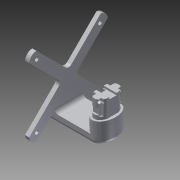
# Autodesk Inventor part: monitor-mount
Saved by Autodesk Inventor 2015 (Build 190159000, 159)
## iProperties
Created: 2015-03-06
Part Number: monitor-mount
Material: ABS Plastic
Document SubType Name: Modeling
Designer: Jody
Density: 1.06 g/cm^3
Appearance: Smooth - White
Mass: 59.874 g
Surface Area: 171.606 cm^2
Volume: 56.4849 cm^3
Author: Jody
Autodesk Inventor part; units mm, degrees
ref_plane "YZ Plane" through (0, 0, 0) normal (1, 0, 0) x (0, 1, 0)
ref_plane "XZ Plane" through (0, 0, 0) normal (0, 1, 0) x (-1, 0, 0)
ref_plane "XY Plane" through (0, 0, 0) normal (0, 0, 1) x (1, 0, 0)
sketch "Sketch1" plane through (0, 0, 0) normal (0, 1, 0) x (-1, 0, 0)
  ellipse E0 centre (0, 0) end of major axis (0, -16.9) minor radius 10.95
  dimension "d0" = 16.9
  dimension "d1" = 10.95
  constraints: 1 coincident, 2 other
extrude "Extrusion1" add sketch "Sketch1" along normal blind 25
sketch "Sketch2" plane through (0, 25, 0) normal (0, 1, 0) x (1, 0, 0)
  line L0 (7.6, 6.869) -> (7.6, -6.8693)
  line L1 (-7.6, -6.8693) -> (-7.6, 6.869)
  line L2 (1.547, -14.35) -> (-1.547, -14.35)
  line L3 (-1.547, 14.35) -> (1.547, 14.35)
  spline S0 degree 5 poles (7.6, 6.869) (7.3339, 7.69) (6.6747, 9.389) (5.6155, 11.3113) (4.2798, 12.863) (2.8086, 13.8602) (1.8557, 14.2496) (1.547, 14.35) knots 0 0 0 0 0 0 0.371815 0.797909 1 1 1 1 1 1
  line L4 (7.9552, 5.7734) -> (7.2448, 7.9647) construction
  arc A0 (7.863, 5.9868) -> (7.2954, 7.7378) centre (-10.8296, 0.8944) ccw construction
  spline S1 degree 5 poles (-1.547, 14.35) (-1.8557, 14.2496) (-2.8086, 13.8602) (-4.2798, 12.863) (-5.6155, 11.3113) (-6.6747, 9.389) (-7.3339, 7.69) (-7.6, 6.869) knots 0 0 0 0 0 0 0.202091 0.628185 1 1 1 1 1 1
  line L5 (-7.2448, 7.9647) -> (-7.9552, 5.7734) construction
  arc A1 (-7.2954, 7.7378) -> (-7.863, 5.9868) centre (10.8296, 0.8944) ccw construction
  spline S2 degree 5 poles (-7.6, -6.8693) (-7.3341, -7.6901) (-6.733, -9.2397) (-5.6943, -11.1801) (-4.3754, -12.7614) (-2.913, -13.7987) (-1.9626, -14.2149) (-1.547, -14.35) knots 0 0 0 0 0 0 0.37178 0.727887 1 1 1 1 1 1
  spline S3 degree 5 poles (1.547, -14.35) (1.9626, -14.2149) (2.913, -13.7987) (4.3754, -12.7614) (5.6943, -11.1801) (6.733, -9.2397) (7.3341, -7.6901) (7.6, -6.8693) knots 0 0 0 0 0 0 0.272113 0.62822 1 1 1 1 1 1
  line L6 (-2.5566, -14.0218) -> (-0.5374, -14.6782) construction
  arc A2 (-2.3246, -14.0283) -> (-0.7288, -14.5471) centre (0.1247, -9.2081) ccw construction
  line L7 (0.5374, -14.6782) -> (2.5566, -14.0218) construction
  arc A3 (0.7288, -14.5471) -> (2.3246, -14.0283) centre (-0.1247, -9.2081) ccw construction
  point P0 (5.4887, -11.1759)
  point P1 (2.672, 13.8453)
  point P2 (-5.4887, 11.1759)
  point P3 (-2.672, -13.8453)
  constraints: 24 end point, 8 midpoint, 4 centre point, 4 point on circle, 2 parallel, 1 horizontal, 1 perpendicular, 24 other
extrude "Extrusion3" add sketch "Sketch2" along normal blind 21
sketch "Sketch6" plane through (0, 46, 0) normal (0, 1, 0) x (1, 0, 0)
  line L0 (3.7, -9.8) -> (10.95, -9.8)
  line L1 (-10.95, -8.35) -> (-3.7, -8.35)
  line L2 (-3.7, -8.35) -> (-3.7, -16.9)
  line L3 (3.7, -9.8) -> (3.7, -16.9)
  line L4 (-3.7, -16.9) -> (-10.95, -8.35)
  line L5 (3.7, -16.9) -> (10.95, -9.8)
  line L6 (3.7, 9.8) -> (10.95, 9.8)
  line L7 (-10.95, 8.35) -> (-3.7, 8.35)
  line L8 (-3.7, 8.35) -> (-3.7, 16.9)
  line L9 (3.7, 9.8) -> (3.7, 16.9)
  line L10 (-3.7, 16.9) -> (-10.95, 8.35)
  line L11 (3.7, 16.9) -> (10.95, 9.8)
  point P0 (0, 0)
  constraints: 24 end point
extrude "Extrusion4" cut sketch "Sketch6" against normal blind 17.7
sketch "Sketch7" plane through (0, 46, 0) normal (0, 1, 0) x (1, 0, 0)
  ellipse E0 centre (0, 0) end of major axis (0, -16.9) minor radius 10.95 projected
  line L0 (10.581, -4.35) -> (-10.581, -4.35)
  line L1 (-10.581, -4.35) -> (-10.581, 4.35)
  line L2 (-10.581, 4.35) -> (10.581, 4.35)
  line L3 (10.581, 4.35) -> (10.581, -4.35)
  line L4 (10.581, -4.35) -> (-10.581, 4.35) construction
  line L5 (-10.581, -4.35) -> (10.581, 4.35) construction
  dimension "d23" = 8.7
  constraints: 12 end point, 2 midpoint, 2 parallel, 1 horizontal, 1 perpendicular, 2 other
  measures "d23" distance of L0.end L1.end
extrude "Extrusion5" cut sketch "Sketch7" against normal blind 2.4 contours L0 L1 L2 L3
sketch "Sketch8" plane through (7.6, 25, 6.8693) normal (1, 0, 0) x (0, 0, -1)
  line L0 (-7.4807, 4.8) -> (-7.4807, 12.1)
  line L1 (-5.4807, 4.8) -> (-5.4807, 12.1)
  line L2 (-7.4807, 4.8) -> (-5.4807, 4.8)
  line L3 (-5.4807, 12.1) -> (-7.4807, 12.1)
  line L4 (21.2193, 4.8) -> (21.2193, 12.1)
  line L5 (19.2193, 4.8) -> (19.2193, 12.1)
  line L6 (21.2193, 4.8) -> (19.2193, 4.8)
  line L7 (19.2193, 12.1) -> (21.2193, 12.1)
  point P0 (6.8693, -25)
  point P1 (0, 0)
  constraints: 16 end point, 2 horizontal
extrude "Extrusion6" cut sketch "Sketch8" against normal up to next
sketch "Sketch9" plane through (-7.6, 25, -6.869) normal (-1, 0, 0) x (0, 0, 1)
  line L0 (3.4692, 5) -> (10.2692, 5)
  line L1 (3.4692, 5) -> (3.4692, 18.6)
  line L2 (10.2692, 5) -> (10.2692, 18.6)
  line L3 (3.4692, 18.6) -> (10.2692, 18.6)
  point P0 (6.869, -25)
  constraints: 8 end point, 1 perpendicular
extrude "Extrusion7" cut sketch "Sketch9" against normal blind 3.5
sketch "Sketch10" plane through (-7.6, 30, -3.3999) normal (0, 0, 1) x (1, 0, 0)
  line L0 (0, 0) -> (3.5, 7.1937)
  line L1 (3.5, 0) -> (3.5, 13.6) projected
  line L2 (3.5, 7.1937) -> (3.5, 8.6937)
  line L3 (3.5, 8.6937) -> (0.864, 10.4946)
  line L4 (0, 0) -> (3.5, 0)
  line L5 (0, 0) -> (3.5, 0) projected
  line L6 (0.864, 10.4946) -> (3.5, 13.6)
  point P0 (7.6, -30)
  dimension "d36" = 8
  dimension "d37" = 1.5
  constraints: 10 end point, 2 point on line, 1 collinear
  measures "d36" distance of L0.start L0.end
  measures "d37" distance of L0.end L2.end
extrude "Extrusion8" add sketch "Sketch10" along normal up to next
fillet "Fillet1" radius 0.5 1 edges at (-6.736, 40.4946, 0.0001)
sketch "Sketch11" plane through (3.7, 46, 13.1272) normal (1, 0, 0) x (0, 0, -1)
  circle A0 centre (1.6989, -3.0978) radius 2.25
  line L0 (17.4772, -2.4) -> (8.7772, -2.4) projected
  line L1 (16.5271, -2.4) -> (9.7271, -2.4) projected
  circle A1 centre (24.5552, -3.0978) radius 2.25
  point P0 (13.1272, -46)
  dimension "d43" = 4.5
  constraints: 2 centre point
  measures "d43" diameter of A0
extrude "Extrusion9" cut sketch "Sketch11" along normal blind 10 and the other way blind 5
sketch "Sketch12" plane through (0, 0, 0) normal (0, -1, 0) x (1, 0, 0)
  ellipse E0 centre (0, 0) end of major axis (0, 16.9) minor radius 10.95 projected
  line L0 (0, 16.9) -> (0, -16.9)
  line L1 (0, -16.9) -> (-50, -16.9)
  line L2 (-50, -16.9) -> (-50, 16.9)
  line L3 (-50, 16.9) -> (0, 16.9)
  dimension "d50" = 50
  constraints: 8 end point, 2 parallel, 1 perpendicular, 1 vertical, 3 other
  measures "d50" distance of L0.end L1.end
extrude "Extrusion10" add sketch "Sketch12" against normal blind 10 contours E0 L1 L2 L3
sketch "Sketch13" plane through (-50, 0, -16.9) normal (-1, 0, 0) x (0, 0, 1)
  circle A0 centre (54.4, 75.1899) radius 2.25
  line L0 (25.3853, 37.6899) -> (63.569, 75.8737)
  line L1 (16.9, 46.1752) -> (55.0838, 84.359)
  arc A1 (63.569, 75.8737) -> (55.0838, 84.359) centre (54.4, 75.1899) ccw
  circle A2 centre (-20.6, 75.1899) radius 2.25
  line L2 (16.9, 46.1752) -> (-21.2838, 84.359)
  line L3 (8.4147, 37.6899) -> (-29.769, 75.8737)
  arc A3 (-21.2838, 84.359) -> (-29.769, 75.8737) centre (-20.6, 75.1899) ccw
  circle A4 centre (54.4, 75.1899) radius 2.25
  line L4 (8.4147, 37.6899) -> (-29.769, -0.4938)
  line L5 (16.9, 29.2046) -> (-21.2838, -8.9791)
  arc A5 (-29.769, -0.4938) -> (-21.2838, -8.9791) centre (-20.6, 0.1899) ccw
  circle A6 centre (54.4, 0.1899) radius 2.25
  line L6 (16.9, 29.2046) -> (55.0838, -8.9791)
  line L7 (25.3853, 37.6899) -> (63.569, -0.4938)
  arc A7 (55.0838, -8.9791) -> (63.569, -0.4938) centre (54.4, 0.1899) ccw
  circle A8 centre (-20.6, 0.1899) radius 2.25
  point P0 (16.9, 37.6899)
  point P1 (16.9, 37.6899)
  point P2 (16.9, 37.6899)
  point P3 (16.9, 37.6899)
  dimension "d58" = 4.5
  dimension "d63" = 4.5
  dimension "d64" = 4.5
  dimension "d65" = 4.5
  dimension "d66" = 4.5
  dimension "d67" = 75
  dimension "d68" = 75
  constraints: 16 end point, 9 centre point, 8 point on circle, 3 coincident
  measures "d58" diameter of A0
  measures "d63" diameter of A2
  measures "d64" diameter of A4
  measures "d65" diameter of A6
  measures "d66" diameter of A8
  measures "d67" distance of A0.centre A2.centre
  measures "d68" distance of A6.centre A1.centre
extrude "Extrusion11" add sketch "Sketch13" against normal blind 5
fillet "Fillet2" radius 5 4 edges at (-47.5, 46.1752, 0) (-47.5, 29.2046, 0) (-47.5, 37.6899, -8.4853) (-47.5, 37.6899, 8.4853)
sketch "Sketch14" plane through (0, 10, 0) normal (0, 1, 0) x (1, 0, 0)
  line L0 (-45, -16.9) -> (-50, -16.9)
  line L1 (-45, 16.9) -> (-45, -16.9)
  line L2 (-45, 16.9) -> (-50, 16.9)
  line L3 (-50, 16.9) -> (-50, -16.9)
  point P0 (0, 0)
  point P1 (-50, 14.2046)
  constraints: 8 end point, 2 horizontal, 2 point on line, 1 perpendicular
extrude "Extrusion12" add sketch "Sketch14" along normal up to next
fillet "Fillet4" radius 5 3 edges at (10.95, 0, 0) (-25, 0, 16.9) (-25, 0, -16.9)
fillet "Fillet5" radius 5 1 edges at (-45, 10, 0)
sketch "Sketch17" plane through (0, 0, 0) normal (0, -1, 0) x (1, 0, 0)
  line L0 (-44, 8.3852) -> (-4.0506, 8.3852) construction
  line L1 (-4.0506, 8.3852) -> (-4.0506, 4) construction
  line L2 (-4.0506, 4) -> (-44, 4) construction
  line L3 (-44, 4) -> (-44, 8.3852) construction
  line L4 (-44, -4.4007) -> (0.0705, -4.4007) construction
  line L5 (0.0705, -4.4007) -> (0.0705, -7.9) construction
  line L6 (0.0705, -7.9) -> (-44, -7.9) construction
  line L7 (-44, -7.9) -> (-44, -4.4007) construction
  line L8 (-50, 11.9) -> (-50, -11.9) projected
  line L9 (0, -11.9) -> (-50, -11.9) projected
  line L10 (-50, 3.5355) -> (-50, -3.5355) projected
  line L11 (-41.6175, 4.7292) -> (-42.06, 4.7292)
  line L12 (-42.06, 4.7292) -> (-42.06, 6.2268)
  spline S0 degree 2 poles (-42.06, 6.2268) (-42.06, 6.4083) (-42.094, 6.7203) (-42.1451, 6.8139) knots 0 0 0 1 2 2 2
  spline S1 degree 2 poles (-42.1451, 6.8139) (-42.1989, 6.9132) (-42.3918, 7.0096) (-42.5563, 7.0096) knots 0 0 0 1 2 2 2
  spline S2 degree 2 poles (-42.5563, 7.0096) (-42.7208, 7.0096) (-43.0697, 6.8338) (-43.237, 6.6919) knots 0 0 0 1 2 2 2
  line L13 (-43.237, 6.6919) -> (-43.237, 4.7292)
  line L14 (-43.237, 4.7292) -> (-43.6795, 4.7292)
  line L15 (-43.6795, 4.7292) -> (-43.6795, 8.3852)
  line L16 (-43.6795, 8.3852) -> (-43.237, 8.3852)
  line L17 (-43.237, 8.3852) -> (-43.237, 7.0635)
  spline S3 degree 2 poles (-43.237, 7.0635) (-43.0385, 7.2422) (-42.6556, 7.4294) (-42.44, 7.4294) knots 0 0 0 1 2 2 2
  spline S4 degree 2 poles (-42.44, 7.4294) (-42.0543, 7.4294) (-41.6175, 6.9188) (-41.6175, 6.4338) knots 0 0 0 1 2 2 2
  line L18 (-41.6175, 6.4338) -> (-41.6175, 4.7292)
  spline S5 degree 2 poles (-40.2022, 4.6782) (-40.5624, 4.6782) (-40.968, 5.0894) (-40.968, 5.5347) knots 0 0 0 1 2 2 2
  line L19 (-40.968, 5.5347) -> (-40.968, 6.9897)
  line L20 (-40.968, 6.9897) -> (-41.2658, 6.9897)
  line L21 (-41.2658, 6.9897) -> (-41.2658, 7.3556)
  line L22 (-41.2658, 7.3556) -> (-40.968, 7.3556)
  line L23 (-40.968, 7.3556) -> (-40.968, 8.1101)
  line L24 (-40.968, 8.1101) -> (-40.5255, 8.1101)
  line L25 (-40.5255, 8.1101) -> (-40.5255, 7.3556)
  line L26 (-40.5255, 7.3556) -> (-39.7115, 7.3556)
  line L27 (-39.7115, 7.3556) -> (-39.7115, 6.9897)
  line L28 (-39.7115, 6.9897) -> (-40.5255, 6.9897)
  line L29 (-40.5255, 6.9897) -> (-40.5255, 5.7389)
  spline S6 degree 2 poles (-40.5255, 5.7389) (-40.5255, 5.5404) (-40.5113, 5.322) (-40.4631, 5.2284) knots 0 0 0 1 2 2 2
  spline S7 degree 2 poles (-40.4631, 5.2284) (-40.4234, 5.1461) (-40.2447, 5.0639) (-40.0916, 5.0639) knots 0 0 0 1 2 2 2
  spline S8 degree 2 poles (-40.0916, 5.0639) (-39.9838, 5.0639) (-39.7824, 5.1291) (-39.737, 5.149) knots 0 0 0 1 2 2 2
  line L30 (-39.737, 5.149) -> (-39.7115, 5.149)
  line L31 (-39.7115, 5.149) -> (-39.7115, 4.7519)
  spline S9 degree 2 poles (-39.7115, 4.7519) (-39.8363, 4.7179) (-40.0916, 4.6782) (-40.2022, 4.6782) knots 0 0 0 1 2 2 2
  spline S10 degree 2 poles (-38.5912, 4.6782) (-38.9514, 4.6782) (-39.357, 5.0894) (-39.357, 5.5347) knots 0 0 0 1 2 2 2
  line L32 (-39.357, 5.5347) -> (-39.357, 6.9897)
  line L33 (-39.357, 6.9897) -> (-39.6548, 6.9897)
  line L34 (-39.6548, 6.9897) -> (-39.6548, 7.3556)
  line L35 (-39.6548, 7.3556) -> (-39.357, 7.3556)
  line L36 (-39.357, 7.3556) -> (-39.357, 8.1101)
  line L37 (-39.357, 8.1101) -> (-38.9145, 8.1101)
  line L38 (-38.9145, 8.1101) -> (-38.9145, 7.3556)
  line L39 (-38.9145, 7.3556) -> (-38.1005, 7.3556)
  line L40 (-38.1005, 7.3556) -> (-38.1005, 6.9897)
  line L41 (-38.1005, 6.9897) -> (-38.9145, 6.9897)
  line L42 (-38.9145, 6.9897) -> (-38.9145, 5.7389)
  spline S11 degree 2 poles (-38.9145, 5.7389) (-38.9145, 5.5404) (-38.9003, 5.322) (-38.8521, 5.2284) knots 0 0 0 1 2 2 2
  spline S12 degree 2 poles (-38.8521, 5.2284) (-38.8124, 5.1461) (-38.6337, 5.0639) (-38.4806, 5.0639) knots 0 0 0 1 2 2 2
  spline S13 degree 2 poles (-38.4806, 5.0639) (-38.3728, 5.0639) (-38.1714, 5.1291) (-38.126, 5.149) knots 0 0 0 1 2 2 2
  line L43 (-38.126, 5.149) -> (-38.1005, 5.149)
  line L44 (-38.1005, 5.149) -> (-38.1005, 4.7519)
  spline S14 degree 2 poles (-38.1005, 4.7519) (-38.2253, 4.7179) (-38.4806, 4.6782) (-38.5912, 4.6782) knots 0 0 0 1 2 2 2
  spline S15 degree 2 poles (-35.5733, 6.1133) (-35.5733, 5.4553) (-36.2002, 4.6782) (-36.6795, 4.6782) knots 0 0 0 1 2 2 2
  spline S16 degree 2 poles (-36.6795, 4.6782) (-36.8752, 4.6782) (-37.1759, 4.7689) (-37.3318, 4.8625) knots 0 0 0 1 2 2 2
  line L45 (-37.3318, 4.8625) -> (-37.3318, 3.762)
  line L46 (-37.3318, 3.762) -> (-37.7743, 3.762)
  line L47 (-37.7743, 3.762) -> (-37.7743, 7.3556)
  line L48 (-37.7743, 7.3556) -> (-37.3318, 7.3556)
  line L49 (-37.3318, 7.3556) -> (-37.3318, 7.0805)
  spline S17 degree 2 poles (-37.3318, 7.0805) (-37.1673, 7.2308) (-36.7646, 7.4294) (-36.5292, 7.4294) knots 0 0 0 1 2 2 2
  spline S18 degree 2 poles (-36.5292, 7.4294) (-36.0782, 7.4294) (-35.5733, 6.7146) (-35.5733, 6.1133) knots 0 0 0 1 2 2 2
  spline S19 degree 2 poles (-36.03, 6.0623) (-36.03, 6.5132) (-36.3165, 7.0096) (-36.637, 7.0096) knots 0 0 0 1 2 2 2
  spline S20 degree 2 poles (-36.637, 7.0096) (-36.8241, 7.0096) (-37.1759, 6.8423) (-37.3318, 6.7118) knots 0 0 0 1 2 2 2
  line L50 (-37.3318, 6.7118) -> (-37.3318, 5.2199)
  spline S21 degree 2 poles (-37.3318, 5.2199) (-37.1588, 5.1376) (-36.9121, 5.0752) (-36.7532, 5.0752) knots 0 0 0 1 2 2 2
  spline S22 degree 2 poles (-36.7532, 5.0752) (-36.41, 5.0752) (-36.03, 5.5801) (-36.03, 6.0623) knots 0 0 0 1 2 2 2
  line L51 (-34.3027, 4.7292) -> (-34.8643, 4.7292)
  line L52 (-34.8643, 4.7292) -> (-34.8643, 5.3986)
  line L53 (-34.8643, 5.3986) -> (-34.3027, 5.3986)
  line L54 (-34.3027, 5.3986) -> (-34.3027, 4.7292)
  line L55 (-34.3027, 6.6863) -> (-34.8643, 6.6863)
  line L56 (-34.8643, 6.6863) -> (-34.8643, 7.3556)
  line L57 (-34.8643, 7.3556) -> (-34.3027, 7.3556)
  line L58 (-34.3027, 7.3556) -> (-34.3027, 6.6863)
  line L59 (-32.0223, 8.3852) -> (-33.3922, 3.9691)
  line L60 (-33.3922, 3.9691) -> (-33.7893, 3.9691)
  line L61 (-33.7893, 3.9691) -> (-32.425, 8.3852)
  line L62 (-32.425, 8.3852) -> (-32.0223, 8.3852)
  line L63 (-30.1815, 8.3852) -> (-31.5515, 3.9691)
  line L64 (-31.5515, 3.9691) -> (-31.9485, 3.9691)
  line L65 (-31.9485, 3.9691) -> (-30.5843, 8.3852)
  line L66 (-30.5843, 8.3852) -> (-30.1815, 8.3852)
  spline S23 degree 2 poles (-27.5721, 6.0424) (-27.5721, 5.3787) (-28.2103, 4.6555) (-28.7435, 4.6555) knots 0 0 0 1 2 2 2
  spline S24 degree 2 poles (-28.7435, 4.6555) (-29.2909, 4.6555) (-29.9177, 5.4014) (-29.9177, 6.0424) knots 0 0 0 1 2 2 2
  spline S25 degree 2 poles (-29.9177, 6.0424) (-29.9177, 6.7004) (-29.2711, 7.4294) (-28.7435, 7.4294) knots 0 0 0 1 2 2 2
  spline S26 degree 2 poles (-28.7435, 7.4294) (-28.2103, 7.4294) (-27.5721, 6.7033) (-27.5721, 6.0424) knots 0 0 0 1 2 2 2
  spline S27 degree 2 poles (-28.0288, 6.0424) (-28.0288, 6.553) (-28.4003, 7.0493) (-28.7435, 7.0493) knots 0 0 0 1 2 2 2
  spline S28 degree 2 poles (-28.7435, 7.0493) (-29.0867, 7.0493) (-29.4611, 6.553) (-29.4611, 6.0424) knots 0 0 0 1 2 2 2
  spline S29 degree 2 poles (-29.4611, 6.0424) (-29.4611, 5.5461) (-29.0867, 5.0355) (-28.7435, 5.0355) knots 0 0 0 1 2 2 2
  spline S30 degree 2 poles (-28.7435, 5.0355) (-28.4032, 5.0355) (-28.0288, 5.5376) (-28.0288, 6.0424) knots 0 0 0 1 2 2 2
  line L67 (-23.936, 7.3556) -> (-24.6025, 4.7292)
  line L68 (-24.6025, 4.7292) -> (-25.0109, 4.7292)
  line L69 (-25.0109, 4.7292) -> (-25.6519, 6.7543)
  line L70 (-25.6519, 6.7543) -> (-26.2901, 4.7292)
  line L71 (-26.2901, 4.7292) -> (-26.6957, 4.7292)
  line L72 (-26.6957, 4.7292) -> (-27.3679, 7.3556)
  line L73 (-27.3679, 7.3556) -> (-26.9084, 7.3556)
  line L74 (-26.9084, 7.3556) -> (-26.4433, 5.322)
  line L75 (-26.4433, 5.322) -> (-25.8221, 7.3556)
  line L76 (-25.8221, 7.3556) -> (-25.4562, 7.3556)
  line L77 (-25.4562, 7.3556) -> (-24.8181, 5.322)
  line L78 (-24.8181, 5.322) -> (-24.3813, 7.3556)
  line L79 (-24.3813, 7.3556) -> (-23.936, 7.3556)
  line L80 (-22.861, 4.7292) -> (-23.4226, 4.7292)
  line L81 (-23.4226, 4.7292) -> (-23.4226, 5.3986)
  line L82 (-23.4226, 5.3986) -> (-22.861, 5.3986)
  line L83 (-22.861, 5.3986) -> (-22.861, 4.7292)
  line L84 (-21.6386, 4.7292) -> (-22.081, 4.7292)
  line L85 (-22.081, 4.7292) -> (-22.081, 8.3852)
  line L86 (-22.081, 8.3852) -> (-21.6386, 8.3852)
  line L87 (-21.6386, 8.3852) -> (-21.6386, 4.7292)
  line L88 (-18.9271, 7.3556) -> (-20.3395, 3.762)
  line L89 (-20.3395, 3.762) -> (-20.8132, 3.762)
  line L90 (-20.8132, 3.762) -> (-20.3424, 4.8568)
  line L91 (-20.3424, 4.8568) -> (-21.2954, 7.3556)
  line L92 (-21.2954, 7.3556) -> (-20.8189, 7.3556)
  line L93 (-20.8189, 7.3556) -> (-20.1013, 5.4099)
  line L94 (-20.1013, 5.4099) -> (-19.3865, 7.3556)
  line L95 (-19.3865, 7.3556) -> (-18.9271, 7.3556)
  line L96 (-17.2026, 8.3852) -> (-18.5725, 3.9691)
  line L97 (-18.5725, 3.9691) -> (-18.9696, 3.9691)
  line L98 (-18.9696, 3.9691) -> (-17.6053, 8.3852)
  line L99 (-17.6053, 8.3852) -> (-17.2026, 8.3852)
  line L100 (-14.1649, 4.7292) -> (-14.769, 4.7292)
  line L101 (-14.769, 4.7292) -> (-16.0482, 6.3573)
  line L102 (-16.0482, 6.3573) -> (-16.2524, 6.1275)
  line L103 (-16.2524, 6.1275) -> (-16.2524, 4.7292)
  line L104 (-16.2524, 4.7292) -> (-16.7176, 4.7292)
  line L105 (-16.7176, 4.7292) -> (-16.7176, 8.2292)
  line L106 (-16.7176, 8.2292) -> (-16.2524, 8.2292)
  line L107 (-16.2524, 8.2292) -> (-16.2524, 6.621)
  line L108 (-16.2524, 6.621) -> (-14.8173, 8.2292)
  line L109 (-14.8173, 8.2292) -> (-14.25, 8.2292)
  line L110 (-14.25, 8.2292) -> (-15.6994, 6.6664)
  line L111 (-15.6994, 6.6664) -> (-14.1649, 4.7292)
  line L112 (-11.8278, 4.7292) -> (-13.9862, 4.7292)
  line L113 (-13.9862, 4.7292) -> (-13.9862, 5.2256)
  spline S31 degree 2 poles (-13.9862, 5.2256) (-13.7536, 5.444) (-13.3395, 5.8496) (-13.141, 6.0679) knots 0 0 0 1 2 2 2
  spline S32 degree 2 poles (-13.141, 6.0679) (-12.7411, 6.5076) (-12.4489, 7.0351) (-12.4489, 7.3159) knots 0 0 0 1 2 2 2
  spline S33 degree 2 poles (-12.4489, 7.3159) (-12.4489, 7.4634) (-12.5397, 7.6846) (-12.622, 7.7555) knots 0 0 0 1 2 2 2
  spline S34 degree 2 poles (-12.622, 7.7555) (-12.7042, 7.8265) (-12.9198, 7.8974) (-13.0502, 7.8974) knots 0 0 0 1 2 2 2
  spline S35 degree 2 poles (-13.0502, 7.8974) (-13.175, 7.8974) (-13.4303, 7.835) (-13.5466, 7.7867) knots 0 0 0 1 2 2 2
  spline S36 degree 2 poles (-13.5466, 7.7867) (-13.6459, 7.747) (-13.8302, 7.6336) (-13.887, 7.5939) knots 0 0 0 1 2 2 2
  line L114 (-13.887, 7.5939) -> (-13.9125, 7.5939)
  line L115 (-13.9125, 7.5939) -> (-13.9125, 8.0931)
  spline S37 degree 2 poles (-13.9125, 8.0931) (-13.7678, 8.164) (-13.2488, 8.303) (-13.0162, 8.303) knots 0 0 0 1 2 2 2
  spline S38 degree 2 poles (-13.0162, 8.303) (-12.5255, 8.303) (-11.9724, 7.7839) (-11.9724, 7.3414) knots 0 0 0 1 2 2 2
  spline S39 degree 2 poles (-11.9724, 7.3414) (-11.9724, 7.1344) (-12.0689, 6.7884) (-12.154, 6.6409) knots 0 0 0 1 2 2 2
  spline S40 degree 2 poles (-12.154, 6.6409) (-12.2391, 6.4877) (-12.4858, 6.1871) (-12.622, 6.0424) knots 0 0 0 1 2 2 2
  spline S41 degree 2 poles (-12.622, 6.0424) (-12.8432, 5.8013) (-13.3849, 5.2851) (-13.5466, 5.1348) knots 0 0 0 1 2 2 2
  line L116 (-13.5466, 5.1348) -> (-11.8278, 5.1348)
  line L117 (-11.8278, 5.1348) -> (-11.8278, 4.7292)
  spline S42 degree 2 poles (-10.2508, 4.6697) (-10.5231, 4.6697) (-10.9741, 4.837) (-11.1357, 5.0072) knots 0 0 0 1 2 2 2
  spline S43 degree 2 poles (-11.1357, 5.0072) (-11.2974, 5.1745) (-11.4761, 5.6907) (-11.4761, 6.0367) knots 0 0 0 1 2 2 2
  spline S44 degree 2 poles (-11.4761, 6.0367) (-11.4761, 6.3828) (-11.2917, 6.8876) (-11.1357, 7.0578) knots 0 0 0 1 2 2 2
  spline S45 degree 2 poles (-11.1357, 7.0578) (-10.9797, 7.2308) (-10.5174, 7.4152) (-10.2508, 7.4152) knots 0 0 0 1 2 2 2
  spline S46 degree 2 poles (-10.2508, 7.4152) (-10.0353, 7.4152) (-9.6325, 7.2932) (-9.4765, 7.2138) knots 0 0 0 1 2 2 2
  line L118 (-9.4765, 7.2138) -> (-9.4765, 6.7175)
  line L119 (-9.4765, 6.7175) -> (-9.502, 6.7175)
  spline S47 degree 2 poles (-9.502, 6.7175) (-9.5502, 6.7572) (-9.6977, 6.8593) (-9.8027, 6.9132) knots 0 0 0 1 2 2 2
  spline S48 degree 2 poles (-9.8027, 6.9132) (-9.8963, 6.9585) (-10.1459, 7.0295) (-10.2593, 7.0295) knots 0 0 0 1 2 2 2
  spline S49 degree 2 poles (-10.2593, 7.0295) (-10.6025, 7.0295) (-11.0194, 6.5104) (-11.0194, 6.0367) knots 0 0 0 1 2 2 2
  spline S50 degree 2 poles (-11.0194, 6.0367) (-11.0194, 5.5744) (-10.6167, 5.0554) (-10.2593, 5.0554) knots 0 0 0 1 2 2 2
  spline S51 degree 2 poles (-10.2593, 5.0554) (-10.0438, 5.0554) (-9.6524, 5.2341) (-9.502, 5.3731) knots 0 0 0 1 2 2 2
  line L120 (-9.502, 5.3731) -> (-9.4765, 5.3731)
  line L121 (-9.4765, 5.3731) -> (-9.4765, 4.8767)
  spline S52 degree 2 poles (-9.4765, 4.8767) (-9.5417, 4.8455) (-9.7403, 4.7576) (-9.8197, 4.7377) knots 0 0 0 1 2 2 2
  spline S53 degree 2 poles (-9.8197, 4.7377) (-9.9331, 4.7037) (-10.1118, 4.6697) (-10.2508, 4.6697) knots 0 0 0 1 2 2 2
  line L122 (-7.0316, 4.7292) -> (-7.4741, 4.7292)
  line L123 (-7.4741, 4.7292) -> (-7.4741, 5.0185)
  spline S54 degree 2 poles (-7.4741, 5.0185) (-7.6783, 4.8398) (-8.0442, 4.6555) (-8.2711, 4.6555) knots 0 0 0 1 2 2 2
  spline S55 degree 2 poles (-8.2711, 4.6555) (-8.4412, 4.6555) (-8.7447, 4.7689) (-8.8553, 4.8909) knots 0 0 0 1 2 2 2
  spline S56 degree 2 poles (-8.8553, 4.8909) (-8.9688, 5.0128) (-9.0936, 5.3844) (-9.0936, 5.651) knots 0 0 0 1 2 2 2
  line L124 (-9.0936, 5.651) -> (-9.0936, 7.3556)
  line L125 (-9.0936, 7.3556) -> (-8.6511, 7.3556)
  line L126 (-8.6511, 7.3556) -> (-8.6511, 5.8581)
  spline S57 degree 2 poles (-8.6511, 5.8581) (-8.6511, 5.6482) (-8.6199, 5.3731) (-8.566, 5.2709) knots 0 0 0 1 2 2 2
  spline S58 degree 2 poles (-8.566, 5.2709) (-8.5122, 5.1688) (-8.3278, 5.0752) (-8.1548, 5.0752) knots 0 0 0 1 2 2 2
  spline S59 degree 2 poles (-8.1548, 5.0752) (-7.9931, 5.0752) (-7.6272, 5.2596) (-7.4741, 5.3929) knots 0 0 0 1 2 2 2
  line L127 (-7.4741, 5.3929) -> (-7.4741, 7.3556)
  line L128 (-7.4741, 7.3556) -> (-7.0316, 7.3556)
  line L129 (-7.0316, 7.3556) -> (-7.0316, 4.7292)
  spline S60 degree 2 poles (-6.297, 4.3094) (-6.2516, 4.2896) (-6.0786, 4.2272) (-5.968, 4.2017) knots 0 0 0 1 2 2 2
  spline S61 degree 2 poles (-5.968, 4.2017) (-5.846, 4.1705) (-5.639, 4.1336) (-5.517, 4.1336) knots 0 0 0 1 2 2 2
  spline S62 degree 2 poles (-5.517, 4.1336) (-5.3128, 4.1336) (-5.0292, 4.2414) (-4.9498, 4.3378) knots 0 0 0 1 2 2 2
  spline S63 degree 2 poles (-4.9498, 4.3378) (-4.8732, 4.4342) (-4.8136, 4.6867) (-4.8136, 4.8483) knots 0 0 0 1 2 2 2
  line L130 (-4.8136, 4.8483) -> (-4.8136, 5.0781)
  spline S64 degree 2 poles (-4.8136, 5.0781) (-4.9923, 4.9221) (-5.3355, 4.7746) (-5.5936, 4.7746) knots 0 0 0 1 2 2 2
  spline S65 degree 2 poles (-5.5936, 4.7746) (-6.0417, 4.7746) (-6.5721, 5.4411) (-6.5721, 6.0679) knots 0 0 0 1 2 2 2
  spline S66 degree 2 poles (-6.5721, 6.0679) (-6.5721, 6.3941) (-6.3878, 6.899) (-6.2346, 7.0777) knots 0 0 0 1 2 2 2
  spline S67 degree 2 poles (-6.2346, 7.0777) (-6.0871, 7.245) (-5.6815, 7.4294) (-5.466, 7.4294) knots 0 0 0 1 2 2 2
  spline S68 degree 2 poles (-5.466, 7.4294) (-5.2618, 7.4294) (-4.9639, 7.3329) (-4.8136, 7.245) knots 0 0 0 1 2 2 2
  line L131 (-4.8136, 7.245) -> (-4.7881, 7.3556)
  line L132 (-4.7881, 7.3556) -> (-4.3712, 7.3556)
  line L133 (-4.3712, 7.3556) -> (-4.3712, 5.0299)
  spline S69 degree 2 poles (-4.3712, 5.0299) (-4.3712, 4.3605) (-4.9526, 3.7365) (-5.5511, 3.7365) knots 0 0 0 1 2 2 2
  spline S70 degree 2 poles (-5.5511, 3.7365) (-5.7439, 3.7365) (-6.1467, 3.7989) (-6.3197, 3.85) knots 0 0 0 1 2 2 2
  line L134 (-6.3197, 3.85) -> (-6.3197, 4.3094)
  line L135 (-6.3197, 4.3094) -> (-6.297, 4.3094)
  line L136 (-4.8136, 5.4411) -> (-4.8136, 6.8848)
  spline S71 degree 2 poles (-4.8136, 6.8848) (-4.9781, 6.9642) (-5.2561, 7.0323) (-5.3951, 7.0323) knots 0 0 0 1 2 2 2
  spline S72 degree 2 poles (-5.3951, 7.0323) (-5.7297, 7.0323) (-6.1155, 6.5388) (-6.1155, 6.0765) knots 0 0 0 1 2 2 2
  spline S73 degree 2 poles (-6.1155, 6.0765) (-6.1155, 5.6397) (-5.8233, 5.183) (-5.4943, 5.183) knots 0 0 0 1 2 2 2
  spline S74 degree 2 poles (-5.4943, 5.183) (-5.3213, 5.183) (-4.9583, 5.3192) (-4.8136, 5.4411) knots 0 0 0 1 2 2 2
  line L137 (-41.0761, -7.5125) -> (-41.4814, -7.5125)
  line L138 (-41.4814, -7.5125) -> (-41.4814, -4.8851)
  line L139 (-41.4814, -4.8851) -> (-42.2773, -6.6721)
  line L140 (-42.2773, -6.6721) -> (-42.5244, -6.6721)
  line L141 (-42.5244, -6.6721) -> (-43.3129, -4.8851)
  line L142 (-43.3129, -4.8851) -> (-43.3129, -7.5125)
  line L143 (-43.3129, -7.5125) -> (-43.691, -7.5125)
  line L144 (-43.691, -7.5125) -> (-43.691, -4.4625)
  line L145 (-43.691, -4.4625) -> (-43.1374, -4.4625)
  line L146 (-43.1374, -4.4625) -> (-42.3761, -6.1605)
  line L147 (-42.3761, -6.1605) -> (-41.6396, -4.4625)
  line L148 (-41.6396, -4.4625) -> (-41.0761, -4.4625)
  line L149 (-41.0761, -4.4625) -> (-41.0761, -7.5125)
  line L150 (-38.2757, -7.5125) -> (-38.7305, -7.5125)
  line L151 (-38.7305, -7.5125) -> (-40.08, -4.8827)
  line L152 (-40.08, -4.8827) -> (-40.08, -7.5125)
  line L153 (-40.08, -7.5125) -> (-40.4581, -7.5125)
  line L154 (-40.4581, -7.5125) -> (-40.4581, -4.4625)
  line L155 (-40.4581, -4.4625) -> (-39.8823, -4.4625)
  line L156 (-39.8823, -4.4625) -> (-38.6538, -6.8773)
  line L157 (-38.6538, -6.8773) -> (-38.6538, -4.4625)
  line L158 (-38.6538, -4.4625) -> (-38.2757, -4.4625)
  line L159 (-38.2757, -4.4625) -> (-38.2757, -7.5125)
  line L160 (-36.9459, -7.5125) -> (-36.9459, -4.8233)
  line L161 (-36.9459, -4.8233) -> (-37.9692, -4.8233)
  line L162 (-37.9692, -4.8233) -> (-37.9692, -4.4625)
  line L163 (-37.9692, -4.4625) -> (-35.5173, -4.4625)
  line L164 (-35.5173, -4.4625) -> (-35.5173, -4.8233)
  line L165 (-35.5173, -4.8233) -> (-36.5406, -4.8233)
  line L166 (-36.5406, -4.8233) -> (-36.5406, -7.5125)
  line L167 (-36.5406, -7.5125) -> (-36.9459, -7.5125)
  line L168 (-34.1777, -6.3632) -> (-35.332, -6.3632)
  line L169 (-35.332, -6.3632) -> (-35.332, -5.9924)
  line L170 (-35.332, -5.9924) -> (-34.1777, -5.9924)
  line L171 (-34.1777, -5.9924) -> (-34.1777, -6.3632)
  spline S75 degree 2 poles (-32.8356, -7.5669) (-33.1668, -7.5669) (-33.6315, -7.4284) (-33.8366, -7.3296) knots 0 0 0 1 2 2 2
  line L172 (-33.8366, -7.3296) -> (-33.8366, -6.8204)
  line L173 (-33.8366, -6.8204) -> (-33.807, -6.8204)
  spline S76 degree 2 poles (-33.807, -6.8204) (-33.6068, -7.0083) (-33.1001, -7.2159) (-32.8653, -7.2159) knots 0 0 0 1 2 2 2
  spline S77 degree 2 poles (-32.8653, -7.2159) (-32.5291, -7.2159) (-32.1856, -6.9366) (-32.1856, -6.7067) knots 0 0 0 1 2 2 2
  spline S78 degree 2 poles (-32.1856, -6.7067) (-32.1856, -6.5238) (-32.366, -6.2964) (-32.5613, -6.2396) knots 0 0 0 1 2 2 2
  spline S79 degree 2 poles (-32.5613, -6.2396) (-32.7021, -6.2) (-32.937, -6.1457) (-33.1124, -6.1012) knots 0 0 0 1 2 2 2
  spline S80 degree 2 poles (-33.1124, -6.1012) (-33.2706, -6.0592) (-33.5203, -5.9331) (-33.6167, -5.8318) knots 0 0 0 1 2 2 2
  spline S81 degree 2 poles (-33.6167, -5.8318) (-33.7106, -5.7304) (-33.8144, -5.4585) (-33.8144, -5.2806) knots 0 0 0 1 2 2 2
  spline S82 degree 2 poles (-33.8144, -5.2806) (-33.8144, -4.9098) (-33.236, -4.4081) (-32.7887, -4.4081) knots 0 0 0 1 2 2 2
  spline S83 degree 2 poles (-32.7887, -4.4081) (-32.5316, -4.4081) (-32.0768, -4.5094) (-31.8816, -4.6058) knots 0 0 0 1 2 2 2
  line L174 (-31.8816, -4.6058) -> (-31.8816, -5.0903)
  line L175 (-31.8816, -5.0903) -> (-31.9112, -5.0903)
  spline S84 degree 2 poles (-31.9112, -5.0903) (-32.057, -4.9568) (-32.5118, -4.7591) (-32.7615, -4.7591) knots 0 0 0 1 2 2 2
  spline S85 degree 2 poles (-32.7615, -4.7591) (-33.0432, -4.7591) (-33.3917, -5.0235) (-33.3917, -5.2386) knots 0 0 0 1 2 2 2
  spline S86 degree 2 poles (-33.3917, -5.2386) (-33.3917, -5.4314) (-33.1866, -5.6612) (-32.9938, -5.7131) knots 0 0 0 1 2 2 2
  spline S87 degree 2 poles (-32.9938, -5.7131) (-32.8653, -5.7477) (-32.4921, -5.8367) (-32.3685, -5.8738) knots 0 0 0 1 2 2 2
  spline S88 degree 2 poles (-32.3685, -5.8738) (-32.0546, -5.9702) (-31.7629, -6.3582) (-31.7629, -6.6425) knots 0 0 0 1 2 2 2
  spline S89 degree 2 poles (-31.7629, -6.6425) (-31.7629, -6.8229) (-31.9088, -7.1689) (-32.0397, -7.29) knots 0 0 0 1 2 2 2
  spline S90 degree 2 poles (-32.0397, -7.29) (-32.1856, -7.4235) (-32.5563, -7.5669) (-32.8356, -7.5669) knots 0 0 0 1 2 2 2
  spline S91 degree 2 poles (-29.5385, -5.9875) (-29.5385, -6.8081) (-30.0155, -7.5767) (-30.5123, -7.5767) knots 0 0 0 1 2 2 2
  spline S92 degree 2 poles (-30.5123, -7.5767) (-31.0165, -7.5767) (-31.4886, -6.7932) (-31.4886, -5.9899) knots 0 0 0 1 2 2 2
  spline S93 degree 2 poles (-31.4886, -5.9899) (-31.4886, -5.1644) (-31.0115, -4.4007) (-30.5123, -4.4007) knots 0 0 0 1 2 2 2
  spline S94 degree 2 poles (-30.5123, -4.4007) (-30.0105, -4.4007) (-29.5385, -5.1916) (-29.5385, -5.9875) knots 0 0 0 1 2 2 2
  spline S95 degree 2 poles (-30.0624, -6.9168) (-30.0031, -6.766) (-29.9537, -6.3014) (-29.9537, -5.9875) knots 0 0 0 1 2 2 2
  spline S96 degree 2 poles (-29.9537, -5.9875) (-29.9537, -5.6736) (-30.0031, -5.2114) (-30.0649, -5.0557) knots 0 0 0 1 2 2 2
  spline S97 degree 2 poles (-30.0649, -5.0557) (-30.1267, -4.9) (-30.3417, -4.7393) (-30.5123, -4.7393) knots 0 0 0 1 2 2 2
  spline S98 degree 2 poles (-30.5123, -4.7393) (-30.6828, -4.7393) (-30.9028, -4.9) (-30.9671, -5.0606) knots 0 0 0 1 2 2 2
  spline S99 degree 2 poles (-30.9671, -5.0606) (-31.0288, -5.2163) (-31.0733, -5.6909) (-31.0733, -5.9899) knots 0 0 0 1 2 2 2
  spline S100 degree 2 poles (-31.0733, -5.9899) (-31.0733, -6.3113) (-31.0338, -6.7413) (-30.9695, -6.9094) knots 0 0 0 1 2 2 2
  spline S101 degree 2 poles (-30.9695, -6.9094) (-30.9102, -7.0676) (-30.6902, -7.2381) (-30.5123, -7.2381) knots 0 0 0 1 2 2 2
  spline S102 degree 2 poles (-30.5123, -7.2381) (-30.3442, -7.2381) (-30.1242, -7.0775) (-30.0624, -6.9168) knots 0 0 0 1 2 2 2
  line L176 (-27.4203, -7.5125) -> (-28.9082, -7.5125)
  line L177 (-28.9082, -7.5125) -> (-28.9082, -7.2011)
  line L178 (-28.9082, -7.2011) -> (-28.3545, -7.2011)
  line L179 (-28.3545, -7.2011) -> (-28.3545, -5.157)
  line L180 (-28.3545, -5.157) -> (-28.9082, -5.157)
  line L181 (-28.9082, -5.157) -> (-28.9082, -4.8777)
  spline S103 degree 2 poles (-28.9082, -4.8777) (-28.5943, -4.8777) (-28.2977, -4.6998) (-28.2779, -4.4526) knots 0 0 0 1 2 2 2
  line L182 (-28.2779, -4.4526) -> (-27.9615, -4.4526)
  line L183 (-27.9615, -4.4526) -> (-27.9615, -7.2011)
  line L184 (-27.9615, -7.2011) -> (-27.4203, -7.2011)
  line L185 (-27.4203, -7.2011) -> (-27.4203, -7.5125)
  line L186 (-25.742, -6.3632) -> (-26.8963, -6.3632)
  line L187 (-26.8963, -6.3632) -> (-26.8963, -5.9924)
  line L188 (-26.8963, -5.9924) -> (-25.742, -5.9924)
  line L189 (-25.742, -5.9924) -> (-25.742, -6.3632)
  line L190 (-23.4212, -4.9197) -> (-24.741, -7.5125)
  line L191 (-24.741, -7.5125) -> (-25.176, -7.5125)
  line L192 (-25.176, -7.5125) -> (-23.782, -4.8209)
  line L193 (-23.782, -4.8209) -> (-25.3564, -4.8209)
  line L194 (-25.3564, -4.8209) -> (-25.3564, -4.4625)
  line L195 (-25.3564, -4.4625) -> (-23.4212, -4.4625)
  line L196 (-23.4212, -4.4625) -> (-23.4212, -4.9197)
  spline S104 degree 2 poles (-21.1991, -6.5436) (-21.1991, -6.7636) (-21.34, -7.1393) (-21.4686, -7.2777) knots 0 0 0 1 2 2 2
  spline S105 degree 2 poles (-21.4686, -7.2777) (-21.5971, -7.4161) (-21.9802, -7.5767) (-22.2175, -7.5767) knots 0 0 0 1 2 2 2
  spline S106 degree 2 poles (-22.2175, -7.5767) (-22.435, -7.5767) (-22.8601, -7.4803) (-23.0158, -7.4037) knots 0 0 0 1 2 2 2
  line L197 (-23.0158, -7.4037) -> (-23.0158, -6.9712)
  line L198 (-23.0158, -6.9712) -> (-22.9861, -6.9712)
  spline S107 degree 2 poles (-22.9861, -6.9712) (-22.9392, -7.0058) (-22.7637, -7.0948) (-22.6574, -7.1343) knots 0 0 0 1 2 2 2
  spline S108 degree 2 poles (-22.6574, -7.1343) (-22.5363, -7.1763) (-22.3361, -7.2233) (-22.21, -7.2233) knots 0 0 0 1 2 2 2
  spline S109 degree 2 poles (-22.21, -7.2233) (-22.0865, -7.2233) (-21.8541, -7.1343) (-21.7701, -7.0379) knots 0 0 0 1 2 2 2
  spline S110 degree 2 poles (-21.7701, -7.0379) (-21.6935, -6.9465) (-21.6144, -6.7043) (-21.6144, -6.5411) knots 0 0 0 1 2 2 2
  spline S111 degree 2 poles (-21.6144, -6.5411) (-21.6144, -6.378) (-21.7034, -6.1704) (-21.7874, -6.1012) knots 0 0 0 1 2 2 2
  spline S112 degree 2 poles (-21.7874, -6.1012) (-21.8739, -6.0246) (-22.131, -5.9603) (-22.2867, -5.9603) knots 0 0 0 1 2 2 2
  spline S113 degree 2 poles (-22.2867, -5.9603) (-22.4547, -5.9603) (-22.7884, -6.0122) (-22.8897, -6.0344) knots 0 0 0 1 2 2 2
  line L199 (-22.8897, -6.0344) -> (-22.8897, -4.4625)
  line L200 (-22.8897, -4.4625) -> (-21.2165, -4.4625)
  line L201 (-21.2165, -4.4625) -> (-21.2165, -4.8209)
  line L202 (-21.2165, -4.8209) -> (-22.4968, -4.8209)
  line L203 (-22.4968, -4.8209) -> (-22.4968, -5.634)
  spline S114 degree 2 poles (-22.4968, -5.634) (-22.4226, -5.6241) (-22.2793, -5.6167) (-22.2199, -5.6167) knots 0 0 0 1 2 2 2
  spline S115 degree 2 poles (-22.2199, -5.6167) (-21.9851, -5.6167) (-21.6613, -5.6934) (-21.513, -5.807) knots 0 0 0 1 2 2 2
  spline S116 degree 2 poles (-21.513, -5.807) (-21.3623, -5.9207) (-21.1991, -6.2668) (-21.1991, -6.5436) knots 0 0 0 1 2 2 2
  line L204 (-18.0577, -7.5125) -> (-18.463, -7.5125)
  line L205 (-18.463, -7.5125) -> (-18.463, -4.8851)
  line L206 (-18.463, -4.8851) -> (-19.2589, -6.6721)
  line L207 (-19.2589, -6.6721) -> (-19.5061, -6.6721)
  line L208 (-19.5061, -6.6721) -> (-20.2945, -4.8851)
  line L209 (-20.2945, -4.8851) -> (-20.2945, -7.5125)
  line L210 (-20.2945, -7.5125) -> (-20.6727, -7.5125)
  line L211 (-20.6727, -7.5125) -> (-20.6727, -4.4625)
  line L212 (-20.6727, -4.4625) -> (-20.119, -4.4625)
  line L213 (-20.119, -4.4625) -> (-19.3578, -6.1605)
  line L214 (-19.3578, -6.1605) -> (-18.6212, -4.4625)
  line L215 (-18.6212, -4.4625) -> (-18.0577, -4.4625)
  line L216 (-18.0577, -4.4625) -> (-18.0577, -7.5125)
  line L217 (-14.8248, -7.5125) -> (-15.2301, -7.5125)
  line L218 (-15.2301, -7.5125) -> (-15.2301, -4.8851)
  line L219 (-15.2301, -4.8851) -> (-16.026, -6.6721)
  line L220 (-16.026, -6.6721) -> (-16.2732, -6.6721)
  line L221 (-16.2732, -6.6721) -> (-17.0616, -4.8851)
  line L222 (-17.0616, -4.8851) -> (-17.0616, -7.5125)
  line L223 (-17.0616, -7.5125) -> (-17.4398, -7.5125)
  line L224 (-17.4398, -7.5125) -> (-17.4398, -4.4625)
  line L225 (-17.4398, -4.4625) -> (-16.8861, -4.4625)
  line L226 (-16.8861, -4.4625) -> (-16.1249, -6.1605)
  line L227 (-16.1249, -6.1605) -> (-15.3883, -4.4625)
  line L228 (-15.3883, -4.4625) -> (-14.8248, -4.4625)
  line L229 (-14.8248, -4.4625) -> (-14.8248, -7.5125)
  line L230 (-11.1297, -5.2237) -> (-11.9923, -7.5125)
  line L231 (-11.9923, -7.5125) -> (-12.3383, -7.5125)
  line L232 (-12.3383, -7.5125) -> (-13.1935, -5.2237)
  line L233 (-13.1935, -5.2237) -> (-12.7758, -5.2237)
  line L234 (-12.7758, -5.2237) -> (-12.1505, -6.986)
  line L235 (-12.1505, -6.986) -> (-11.5301, -5.2237)
  line L236 (-11.5301, -5.2237) -> (-11.1297, -5.2237)
  line L237 (-9.1672, -7.5125) -> (-10.6551, -7.5125)
  line L238 (-10.6551, -7.5125) -> (-10.6551, -7.2011)
  line L239 (-10.6551, -7.2011) -> (-10.1015, -7.2011)
  line L240 (-10.1015, -7.2011) -> (-10.1015, -5.157)
  line L241 (-10.1015, -5.157) -> (-10.6551, -5.157)
  line L242 (-10.6551, -5.157) -> (-10.6551, -4.8777)
  spline S117 degree 2 poles (-10.6551, -4.8777) (-10.3412, -4.8777) (-10.0447, -4.6998) (-10.0249, -4.4526) knots 0 0 0 1 2 2 2
  line L243 (-10.0249, -4.4526) -> (-9.7085, -4.4526)
  line L244 (-9.7085, -4.4526) -> (-9.7085, -7.2011)
  line L245 (-9.7085, -7.2011) -> (-9.1672, -7.2011)
  line L246 (-9.1672, -7.2011) -> (-9.1672, -7.5125)
  dimension "d80" = 6
  dimension "d81" = 6
  dimension "d82" = 4
  constraints: 4 other
  measures "d80" distance from line of L8 L0.start
  measures "d81" distance from line of L8 L4.start
  measures "d82" distance from line of L9 L6.end
extrude "Extrusion13" cut sketch "Sketch17" against normal blind 0.5
body "Solid1"
